Autodesk Inventor part; units mm, degrees
(part 4 of 6)
  line L840 (29.0828, -25.8646) -> (29.0171, -26.0875) projected
  line L841 (29.1718, -25.6412) -> (29.0828, -25.8646) projected
  line L842 (29.3021, -25.4012) -> (29.1718, -25.6412) projected
  line L843 (29.5054, -25.1196) -> (29.3021, -25.4012) projected
  line L844 (29.5412, -25.0774) -> (29.5054, -25.1196) projected
  line L845 (29.5771, -25.0351) -> (29.5412, -25.0774) projected
  line L846 (29.6129, -24.9928) -> (29.5771, -25.0351) projected
  line L847 (29.6486, -24.9504) -> (29.6129, -24.9928) projected
  line L848 (29.6842, -24.908) -> (29.6486, -24.9504) projected
  line L849 (29.7198, -24.8655) -> (29.6842, -24.908) projected
  line L850 (29.7553, -24.823) -> (29.7198, -24.8655) projected
  line L851 (29.7908, -24.7804) -> (29.7553, -24.823) projected
  line L852 (29.8262, -24.7378) -> (29.7908, -24.7804) projected
  line L853 (29.8616, -24.6951) -> (29.8262, -24.7378) projected
  line L854 (30.1036, -24.4461) -> (29.8616, -24.6951) projected
  line L855 (30.3173, -24.2761) -> (30.1036, -24.4461) projected
  line L856 (30.5219, -24.1496) -> (30.3173, -24.2761) projected
  line L857 (30.7299, -24.0462) -> (30.5219, -24.1496) projected
  line L858 (30.9366, -23.9692) -> (30.7299, -24.0462) projected
  line L859 (31.1483, -23.9085) -> (30.9366, -23.9692) projected
  line L860 (31.3597, -23.8696) -> (31.1483, -23.9085) projected
  line L861 (31.575, -23.8461) -> (31.3597, -23.8696) projected
  line L862 (31.7918, -23.8401) -> (31.575, -23.8461) projected
  line L863 (32.0092, -23.8521) -> (31.7918, -23.8401) projected
  line L864 (32.231, -23.8765) -> (32.0092, -23.8521) projected
  line L865 (32.4525, -23.9189) -> (32.231, -23.8765) projected
  line L866 (32.6748, -23.9775) -> (32.4525, -23.9189) projected
  line L867 (32.9013, -24.0471) -> (32.6748, -23.9775) projected
  line L868 (33.1282, -24.1326) -> (32.9013, -24.0471) projected
  line L869 (33.3555, -24.2337) -> (33.1282, -24.1326) projected
  line L870 (33.583, -24.3502) -> (33.3555, -24.2337) projected
  line L871 (33.814, -24.4773) -> (33.583, -24.3502) projected
  line L872 (34.0465, -24.6174) -> (33.814, -24.4773) projected
  line L873 (34.2792, -24.772) -> (34.0465, -24.6174) projected
  line L874 (34.6041, -24.9642) -> (34.2792, -24.772) projected
  line L875 (34.9452, -25.1339) -> (34.6041, -24.9642) projected
  line L876 (35.2972, -25.2883) -> (34.9452, -25.1339) projected
  line L877 (35.6581, -25.4299) -> (35.2972, -25.2883) projected
  line L878 (36.0268, -25.5601) -> (35.6581, -25.4299) projected
  line L879 (36.4025, -25.68) -> (36.0268, -25.5601) projected
  line L880 (36.7847, -25.7901) -> (36.4025, -25.68) projected
  line L881 (37.1729, -25.8909) -> (36.7847, -25.7901) projected
  line L882 (37.5667, -25.9828) -> (37.1729, -25.8909) projected
  line L883 (37.9659, -26.0661) -> (37.5667, -25.9828) projected
  line L884 (38.3701, -26.1411) -> (37.9659, -26.0661) projected
  line L885 (38.7791, -26.2078) -> (38.3701, -26.1411) projected
  line L886 (39.1928, -26.2665) -> (38.7791, -26.2078) projected
  line L887 (39.6108, -26.3174) -> (39.1928, -26.2665) projected
  line L888 (40.0331, -26.3604) -> (39.6108, -26.3174) projected
  line L889 (40.4594, -26.3957) -> (40.0331, -26.3604) projected
  line L890 (40.8897, -26.4234) -> (40.4594, -26.3957) projected
  line L891 (41.3237, -26.4435) -> (40.8897, -26.4234) projected
  line L892 (41.7614, -26.4561) -> (41.3237, -26.4435) projected
  line L893 (42.2025, -26.4613) -> (41.7614, -26.4561) projected
  line L894 (42.3943, -26.153) -> (42.2025, -26.4613) projected
  line L895 (42.5838, -25.8433) -> (42.3943, -26.153) projected
  line L896 (42.771, -25.5322) -> (42.5838, -25.8433) projected
  line L897 (42.9559, -25.2198) -> (42.771, -25.5322) projected
  line L898 (43.1386, -24.9061) -> (42.9559, -25.2198) projected
  line L899 (43.319, -24.591) -> (43.1386, -24.9061) projected
  line L900 (43.4971, -24.2746) -> (43.319, -24.591) projected
  line L901 (43.6728, -23.957) -> (43.4971, -24.2746) projected
  line L902 (43.8463, -23.638) -> (43.6728, -23.957) projected
  line L903 (44.0174, -23.3178) -> (43.8463, -23.638) projected
  line L904 (43.7924, -22.9383) -> (44.0174, -23.3178) projected
  line L905 (43.5626, -22.5656) -> (43.7924, -22.9383) projected
  line L906 (43.3282, -22.1998) -> (43.5626, -22.5656) projected
  line L907 (43.0891, -21.841) -> (43.3282, -22.1998) projected
  line L908 (42.8453, -21.4895) -> (43.0891, -21.841) projected
  line L909 (42.5969, -21.1453) -> (42.8453, -21.4895) projected
  line L910 (42.3439, -20.8086) -> (42.5969, -21.1453) projected
  line L911 (42.0862, -20.4798) -> (42.3439, -20.8086) projected
  line L912 (41.8239, -20.1589) -> (42.0862, -20.4798) projected
  line L913 (41.5569, -19.8464) -> (41.8239, -20.1589) projected
  line L914 (41.2851, -19.5423) -> (41.5569, -19.8464) projected
  line L915 (41.0086, -19.2472) -> (41.2851, -19.5423) projected
  line L916 (40.7272, -18.9615) -> (41.0086, -19.2472) projected
  line L917 (40.4408, -18.6855) -> (40.7272, -18.9615) projected
  line L918 (40.1491, -18.4201) -> (40.4408, -18.6855) projected
  line L919 (39.852, -18.1659) -> (40.1491, -18.4201) projected
  line L920 (39.5489, -17.9241) -> (39.852, -18.1659) projected
  line L921 (39.2392, -17.6965) -> (39.5489, -17.9241) projected
  line L922 (38.9217, -17.4859) -> (39.2392, -17.6965) projected
  line L923 (38.5928, -17.3007) -> (38.9217, -17.4859) projected
  line L924 (38.3425, -17.1764) -> (38.5928, -17.3007) projected
  line L925 (38.105, -17.0451) -> (38.3425, -17.1764) projected
  line L926 (37.8794, -16.9086) -> (38.105, -17.0451) projected
  line L927 (37.6648, -16.7698) -> (37.8794, -16.9086) projected
  line L928 (37.4636, -16.6236) -> (37.6648, -16.7698) projected
  line L929 (37.2761, -16.4698) -> (37.4636, -16.6236) projected
  line L930 (37.1025, -16.3084) -> (37.2761, -16.4698) projected
  line L931 (36.9406, -16.1452) -> (37.1025, -16.3084) projected
  line L932 (36.7931, -15.9746) -> (36.9406, -16.1452) projected
  line L933 (36.6611, -15.7947) -> (36.7931, -15.9746) projected
  line L934 (36.5421, -15.6124) -> (36.6611, -15.7947) projected
  line L935 (36.4388, -15.4218) -> (36.5421, -15.6124) projected
  line L936 (36.3516, -15.2235) -> (36.4388, -15.4218) projected
  line L937 (36.2795, -15.0209) -> (36.3516, -15.2235) projected
  line L938 (36.2262, -14.8073) -> (36.2795, -15.0209) projected
  line L939 (36.1896, -14.5898) -> (36.2262, -14.8073) projected
  line L940 (36.1751, -14.3579) -> (36.1896, -14.5898) projected
  line L941 (36.1824, -14.1175) -> (36.1751, -14.3579) projected
  line L942 (36.2227, -13.8474) -> (36.1824, -14.1175) projected
  line L943 (36.3174, -13.5133) -> (36.2227, -13.8474) projected
  line L944 (36.3367, -13.4614) -> (36.3174, -13.5133) projected
  line L945 (36.3559, -13.4094) -> (36.3367, -13.4614) projected
  line L946 (36.375, -13.3574) -> (36.3559, -13.4094) projected
  line L947 (36.3941, -13.3053) -> (36.375, -13.3574) projected
  line L948 (36.4131, -13.2533) -> (36.3941, -13.3053) projected
  line L949 (36.432, -13.2012) -> (36.4131, -13.2533) projected
  line L950 (36.4508, -13.1491) -> (36.432, -13.2012) projected
  line L951 (36.4696, -13.0969) -> (36.4508, -13.1491) projected
  line L952 (36.4883, -13.0448) -> (36.4696, -13.0969) projected
  line L953 (36.5069, -12.9926) -> (36.4883, -13.0448) projected
  line L954 (36.6492, -12.6758) -> (36.5069, -12.9926) projected
  line L955 (36.7919, -12.4429) -> (36.6492, -12.6758) projected
  line L956 (36.9408, -12.2541) -> (36.7919, -12.4429) projected
  line L957 (37.1009, -12.0858) -> (36.9408, -12.2541) projected
  line L958 (37.2688, -11.9427) -> (37.1009, -12.0858) projected
  line L959 (37.447, -11.8133) -> (37.2688, -11.9427) projected
  line L960 (37.6324, -11.7044) -> (37.447, -11.8133) projected
  line L961 (37.8267, -11.6087) -> (37.6324, -11.7044) projected
  line L962 (38.0283, -11.529) -> (37.8267, -11.6087) projected
  line L963 (38.2367, -11.4659) -> (38.0283, -11.529) projected
  line L964 (38.4534, -11.4129) -> (38.2367, -11.4659) projected
  line L965 (38.6761, -11.377) -> (38.4534, -11.4129) projected
  line L966 (38.905, -11.3561) -> (38.6761, -11.377) projected
  line L967 (39.1417, -11.344) -> (38.905, -11.3561) projected
  line L968 (39.3842, -11.3467) -> (39.1417, -11.344) projected
  line L969 (39.6323, -11.364) -> (39.3842, -11.3467) projected
  line L970 (39.886, -11.3956) -> (39.6323, -11.364) projected
  line L971 (40.1465, -11.4361) -> (39.886, -11.3956) projected
  line L972 (40.4129, -11.4882) -> (40.1465, -11.4361) projected
  line L973 (40.6845, -11.5538) -> (40.4129, -11.4882) projected
  line L974 (41.0555, -11.6234) -> (40.6845, -11.5538) projected
  line L975 (41.4341, -11.6662) -> (41.0555, -11.6234) projected
  line L976 (41.8176, -11.6908) -> (41.4341, -11.6662) projected
  line L977 (42.2052, -11.7005) -> (41.8176, -11.6908) projected
  line L978 (42.5962, -11.6968) -> (42.2052, -11.7005) projected
  line L979 (42.9903, -11.6809) -> (42.5962, -11.6968) projected
  line L980 (43.387, -11.6536) -> (42.9903, -11.6809) projected
  line L981 (43.7863, -11.6156) -> (43.387, -11.6536) projected
  line L982 (44.1878, -11.5673) -> (43.7863, -11.6156) projected
  line L983 (44.5914, -11.509) -> (44.1878, -11.5673) projected
  line L984 (44.9969, -11.4412) -> (44.5914, -11.509) projected
  line L985 (45.4041, -11.3641) -> (44.9969, -11.4412) projected
  line L986 (45.8128, -11.2778) -> (45.4041, -11.3641) projected
  line L987 (46.223, -11.1825) -> (45.8128, -11.2778) projected
  line L988 (46.6346, -11.0786) -> (46.223, -11.1825) projected
  line L989 (47.0473, -10.9659) -> (46.6346, -11.0786) projected
  line L990 (47.4611, -10.8448) -> (47.0473, -10.9659) projected
  line L991 (47.8758, -10.7152) -> (47.4611, -10.8448) projected
  line L992 (48.2914, -10.5774) -> (47.8758, -10.7152) projected
  line L993 (48.7077, -10.4313) -> (48.2914, -10.5774) projected
  line L994 (48.7824, -10.0761) -> (48.7077, -10.4313) projected
  line L995 (48.8546, -9.7203) -> (48.7824, -10.0761) projected
  line L996 (48.9241, -9.3639) -> (48.8546, -9.7203) projected
  line L997 (48.9911, -9.0071) -> (48.9241, -9.3639) projected
  line L998 (49.0554, -8.6498) -> (48.9911, -9.0071) projected
  line L999 (49.1172, -8.292) -> (49.0554, -8.6498) projected
  line L1000 (49.1763, -7.9338) -> (49.1172, -8.292) projected
  line L1001 (49.2328, -7.5752) -> (49.1763, -7.9338) projected
  line L1002 (49.2867, -7.2162) -> (49.2328, -7.5752) projected
  line L1003 (49.338, -6.8568) -> (49.2867, -7.2162) projected
  line L1004 (48.9968, -6.5771) -> (49.338, -6.8568) projected
  line L1005 (48.6534, -6.3055) -> (48.9968, -6.5771) projected
  line L1006 (48.308, -6.0419) -> (48.6534, -6.3055) projected
  line L1007 (47.9606, -5.7865) -> (48.308, -6.0419) projected
  line L1008 (47.6113, -5.5395) -> (47.9606, -5.7865) projected
  line L1009 (47.2601, -5.3011) -> (47.6113, -5.5395) projected
  line L1010 (46.9072, -5.0713) -> (47.2601, -5.3011) projected
  line L1011 (46.5526, -4.8504) -> (46.9072, -5.0713) projected
  line L1012 (46.1963, -4.6386) -> (46.5526, -4.8504) projected
  line L1013 (45.8385, -4.4362) -> (46.1963, -4.6386) projected
  line L1014 (45.4792, -4.2434) -> (45.8385, -4.4362) projected
  line L1015 (45.1184, -4.0607) -> (45.4792, -4.2434) projected
  line L1016 (44.7563, -3.8884) -> (45.1184, -4.0607) projected
  line L1017 (44.3927, -3.7271) -> (44.7563, -3.8884) projected
  line L1018 (44.0279, -3.5774) -> (44.3927, -3.7271) projected
  line L1019 (43.6617, -3.4402) -> (44.0279, -3.5774) projected
  line L1020 (43.2942, -3.3167) -> (43.6617, -3.4402) projected
  line L1021 (42.9254, -3.2087) -> (43.2942, -3.3167) projected
  line L1022 (42.555, -3.1194) -> (42.9254, -3.2087) projected
  line L1023 (42.1825, -3.0578) -> (42.555, -3.1194) projected
  line L1024 (41.9049, -3.0266) -> (42.1825, -3.0578) projected
  line L1025 (41.6367, -2.9845) -> (41.9049, -3.0266) projected
  line L1026 (41.3781, -2.9334) -> (41.6367, -2.9845) projected
  line L1027 (41.1289, -2.8764) -> (41.3781, -2.9334) projected
  line L1028 (40.8898, -2.8078) -> (41.1289, -2.8764) projected
  line L1029 (40.661, -2.7274) -> (40.8898, -2.8078) projected
  line L1030 (40.4428, -2.6351) -> (40.661, -2.7274) projected
  line L1031 (40.2348, -2.5371) -> (40.4428, -2.6351) projected
  line L1032 (40.0379, -2.4272) -> (40.2348, -2.5371) projected
  line L1033 (39.8523, -2.3033) -> (40.0379, -2.4272) projected
  line L1034 (39.6781, -2.1727) -> (39.8523, -2.3033) projected
  line L1035 (39.5158, -2.0289) -> (39.6781, -2.1727) projected
  line L1036 (39.366, -1.8725) -> (39.5158, -2.0289) projected
  line L1037 (39.2291, -1.7067) -> (39.366, -1.8725) projected
  line L1038 (39.1059, -1.5242) -> (39.2291, -1.7067) projected
  line L1039 (38.997, -1.3323) -> (39.1059, -1.5242) projected
  line L1040 (38.9042, -1.1194) -> (38.997, -1.3323) projected
  line L1041 (38.8288, -0.891) -> (38.9042, -1.1194) projected
  line L1042 (38.7743, -0.6234) -> (38.8288, -0.891) projected
  line L1043 (38.749, -0.2771) -> (38.7743, -0.6234) projected
  line L1044 (38.7494, -0.2217) -> (38.749, -0.2771) projected
  line L1045 (38.7496, -0.1663) -> (38.7494, -0.2217) projected
  line L1046 (38.7498, -0.1108) -> (38.7496, -0.1663) projected
  line L1047 (38.75, -0.0554) -> (38.7498, -0.1108) projected
  line L1048 (38.75, 0) -> (38.75, -0.0554) projected
  line L1049 (38.75, 0.0554) -> (38.75, 0) projected
  line L1050 (38.7498, 0.1108) -> (38.75, 0.0554) projected
  line L1051 (38.7496, 0.1663) -> (38.7498, 0.1108) projected
  line L1052 (38.7494, 0.2217) -> (38.7496, 0.1663) projected
  line L1053 (38.749, 0.2771) -> (38.7494, 0.2217) projected
  line L1054 (38.7743, 0.6234) -> (38.749, 0.2771) projected
  line L1055 (38.8288, 0.891) -> (38.7743, 0.6234) projected
  line L1056 (38.9042, 1.1194) -> (38.8288, 0.891) projected
  line L1057 (38.997, 1.3323) -> (38.9042, 1.1194) projected
  line L1058 (39.1059, 1.5242) -> (38.997, 1.3323) projected
  line L1059 (39.2291, 1.7067) -> (39.1059, 1.5242) projected
  line L1060 (39.366, 1.8725) -> (39.2291, 1.7067) projected
  line L1061 (39.5158, 2.0289) -> (39.366, 1.8725) projected
  line L1062 (39.6781, 2.1727) -> (39.5158, 2.0289) projected
  line L1063 (39.8523, 2.3033) -> (39.6781, 2.1727) projected
  line L1064 (40.0379, 2.4272) -> (39.8523, 2.3033) projected
  line L1065 (40.2348, 2.5371) -> (40.0379, 2.4272) projected
  line L1066 (40.4428, 2.6351) -> (40.2348, 2.5371) projected
  line L1067 (40.661, 2.7274) -> (40.4428, 2.6351) projected
  line L1068 (40.8898, 2.8078) -> (40.661, 2.7274) projected
  line L1069 (41.1289, 2.8764) -> (40.8898, 2.8078) projected
  line L1070 (41.3781, 2.9334) -> (41.1289, 2.8764) projected
  line L1071 (41.6367, 2.9845) -> (41.3781, 2.9334) projected
  line L1072 (41.9049, 3.0266) -> (41.6367, 2.9845) projected
  line L1073 (42.1825, 3.0578) -> (41.9049, 3.0266) projected
  line L1074 (42.555, 3.1194) -> (42.1825, 3.0578) projected
  line L1075 (42.9254, 3.2087) -> (42.555, 3.1194) projected
  line L1076 (43.2942, 3.3167) -> (42.9254, 3.2087) projected
  line L1077 (43.6617, 3.4402) -> (43.2942, 3.3167) projected
  line L1078 (44.0279, 3.5774) -> (43.6617, 3.4402) projected
  line L1079 (44.3927, 3.7271) -> (44.0279, 3.5774) projected
  line L1080 (44.7563, 3.8884) -> (44.3927, 3.7271) projected
  line L1081 (45.1184, 4.0607) -> (44.7563, 3.8884) projected
  line L1082 (45.4792, 4.2434) -> (45.1184, 4.0607) projected
  line L1083 (45.8385, 4.4362) -> (45.4792, 4.2434) projected
  line L1084 (46.1963, 4.6386) -> (45.8385, 4.4362) projected
  line L1085 (46.5526, 4.8504) -> (46.1963, 4.6386) projected
  line L1086 (46.9072, 5.0713) -> (46.5526, 4.8504) projected
  line L1087 (47.2601, 5.3011) -> (46.9072, 5.0713) projected
  line L1088 (47.6113, 5.5395) -> (47.2601, 5.3011) projected
  line L1089 (47.9606, 5.7865) -> (47.6113, 5.5395) projected
  line L1090 (48.308, 6.0419) -> (47.9606, 5.7865) projected
  line L1091 (48.6534, 6.3055) -> (48.308, 6.0419) projected
  line L1092 (48.9968, 6.5771) -> (48.6534, 6.3055) projected
  line L1093 (49.338, 6.8568) -> (48.9968, 6.5771) projected
  line L1094 (49.2867, 7.2162) -> (49.338, 6.8568) projected
  line L1095 (49.2328, 7.5752) -> (49.2867, 7.2162) projected
  line L1096 (49.1763, 7.9338) -> (49.2328, 7.5752) projected
  line L1097 (49.1172, 8.292) -> (49.1763, 7.9338) projected
  line L1098 (49.0554, 8.6498) -> (49.1172, 8.292) projected
  line L1099 (48.9911, 9.0071) -> (49.0554, 8.6498) projected
  line L1100 (48.9241, 9.3639) -> (48.9911, 9.0071) projected
  line L1101 (48.8546, 9.7203) -> (48.9241, 9.3639) projected
  line L1102 (48.7824, 10.0761) -> (48.8546, 9.7203) projected
  line L1103 (48.7077, 10.4313) -> (48.7824, 10.0761) projected
  line L1104 (48.2914, 10.5774) -> (48.7077, 10.4313) projected
  line L1105 (47.8758, 10.7152) -> (48.2914, 10.5774) projected
  line L1106 (47.4611, 10.8448) -> (47.8758, 10.7152) projected
  line L1107 (47.0473, 10.9659) -> (47.4611, 10.8448) projected
  line L1108 (46.6346, 11.0786) -> (47.0473, 10.9659) projected
  line L1109 (46.223, 11.1825) -> (46.6346, 11.0786) projected
  line L1110 (45.8128, 11.2778) -> (46.223, 11.1825) projected
  line L1111 (45.4041, 11.3641) -> (45.8128, 11.2778) projected
  line L1112 (44.9969, 11.4412) -> (45.4041, 11.3641) projected
  line L1113 (44.5914, 11.509) -> (44.9969, 11.4412) projected
  line L1114 (44.1878, 11.5673) -> (44.5914, 11.509) projected
  line L1115 (43.7863, 11.6156) -> (44.1878, 11.5673) projected
  line L1116 (43.387, 11.6536) -> (43.7863, 11.6156) projected
  line L1117 (42.9903, 11.6809) -> (43.387, 11.6536) projected
  line L1118 (42.5962, 11.6968) -> (42.9903, 11.6809) projected
  line L1119 (42.2052, 11.7005) -> (42.5962, 11.6968) projected
  line L1120 (41.8176, 11.6908) -> (42.2052, 11.7005) projected
  line L1121 (41.4341, 11.6662) -> (41.8176, 11.6908) projected
  line L1122 (41.0555, 11.6234) -> (41.4341, 11.6662) projected
  line L1123 (40.6845, 11.5538) -> (41.0555, 11.6234) projected
  line L1124 (40.4129, 11.4882) -> (40.6845, 11.5538) projected
  line L1125 (40.1465, 11.4361) -> (40.4129, 11.4882) projected
  line L1126 (39.886, 11.3956) -> (40.1465, 11.4361) projected
  line L1127 (39.6323, 11.364) -> (39.886, 11.3956) projected
  line L1128 (39.3842, 11.3467) -> (39.6323, 11.364) projected
  line L1129 (39.1417, 11.344) -> (39.3842, 11.3467) projected
  line L1130 (38.905, 11.3561) -> (39.1417, 11.344) projected
  line L1131 (38.6761, 11.377) -> (38.905, 11.3561) projected
  line L1132 (38.4534, 11.4129) -> (38.6761, 11.377) projected
  line L1133 (38.2367, 11.4659) -> (38.4534, 11.4129) projected
  line L1134 (38.0283, 11.529) -> (38.2367, 11.4659) projected
  line L1135 (37.8267, 11.6087) -> (38.0283, 11.529) projected
  line L1136 (37.6324, 11.7044) -> (37.8267, 11.6087) projected
  line L1137 (37.447, 11.8133) -> (37.6324, 11.7044) projected
  line L1138 (37.2688, 11.9427) -> (37.447, 11.8133) projected
  line L1139 (37.1009, 12.0858) -> (37.2688, 11.9427) projected
  line L1140 (36.9408, 12.2541) -> (37.1009, 12.0858) projected
  line L1141 (36.7919, 12.4429) -> (36.9408, 12.2541) projected
  line L1142 (36.6492, 12.6758) -> (36.7919, 12.4429) projected
  line L1143 (36.5069, 12.9926) -> (36.6492, 12.6758) projected
  line L1144 (36.4883, 13.0448) -> (36.5069, 12.9926) projected
  line L1145 (36.4696, 13.0969) -> (36.4883, 13.0448) projected
  line L1146 (36.4508, 13.1491) -> (36.4696, 13.0969) projected
  line L1147 (36.432, 13.2012) -> (36.4508, 13.1491) projected
  line L1148 (36.4131, 13.2533) -> (36.432, 13.2012) projected
  line L1149 (36.3941, 13.3053) -> (36.4131, 13.2533) projected
  line L1150 (36.375, 13.3574) -> (36.3941, 13.3053) projected
  line L1151 (36.3559, 13.4094) -> (36.375, 13.3574) projected
  line L1152 (36.3367, 13.4614) -> (36.3559, 13.4094) projected
  line L1153 (36.3174, 13.5133) -> (36.3367, 13.4614) projected
  line L1154 (36.2227, 13.8474) -> (36.3174, 13.5133) projected
  line L1155 (36.1824, 14.1175) -> (36.2227, 13.8474) projected
  line L1156 (36.1751, 14.3579) -> (36.1824, 14.1175) projected
  line L1157 (36.1896, 14.5898) -> (36.1751, 14.3579) projected
  line L1158 (36.2262, 14.8073) -> (36.1896, 14.5898) projected
  line L1159 (36.2795, 15.0209) -> (36.2262, 14.8073) projected
  line L1160 (36.3516, 15.2235) -> (36.2795, 15.0209) projected
  line L1161 (36.4388, 15.4218) -> (36.3516, 15.2235) projected
  line L1162 (36.5421, 15.6124) -> (36.4388, 15.4218) projected
  line L1163 (36.6611, 15.7947) -> (36.5421, 15.6124) projected
  line L1164 (36.7931, 15.9746) -> (36.6611, 15.7947) projected
  line L1165 (36.9406, 16.1452) -> (36.7931, 15.9746) projected
  line L1166 (37.1025, 16.3084) -> (36.9406, 16.1452) projected
  line L1167 (37.2761, 16.4698) -> (37.1025, 16.3084) projected
  line L1168 (37.4636, 16.6236) -> (37.2761, 16.4698) projected
  line L1169 (37.6648, 16.7698) -> (37.4636, 16.6236) projected
  line L1170 (37.8794, 16.9086) -> (37.6648, 16.7698) projected
  line L1171 (38.105, 17.0451) -> (37.8794, 16.9086) projected
  line L1172 (38.3425, 17.1764) -> (38.105, 17.0451) projected
  line L1173 (38.5928, 17.3007) -> (38.3425, 17.1764) projected
  line L1174 (38.9217, 17.4859) -> (38.5928, 17.3007) projected
  line L1175 (39.2392, 17.6965) -> (38.9217, 17.4859) projected
  line L1176 (39.5489, 17.9241) -> (39.2392, 17.6965) projected
  line L1177 (39.852, 18.1659) -> (39.5489, 17.9241) projected
  line L1178 (40.1491, 18.4201) -> (39.852, 18.1659) projected
  line L1179 (40.4408, 18.6855) -> (40.1491, 18.4201) projected
  line L1180 (40.7272, 18.9615) -> (40.4408, 18.6855) projected
  line L1181 (41.0086, 19.2472) -> (40.7272, 18.9615) projected
  line L1182 (41.2851, 19.5423) -> (41.0086, 19.2472) projected
  line L1183 (41.5569, 19.8464) -> (41.2851, 19.5423) projected
  line L1184 (41.8239, 20.1589) -> (41.5569, 19.8464) projected
  line L1185 (42.0862, 20.4798) -> (41.8239, 20.1589) projected
  line L1186 (42.3439, 20.8086) -> (42.0862, 20.4798) projected
  line L1187 (42.5969, 21.1453) -> (42.3439, 20.8086) projected
  line L1188 (42.8453, 21.4895) -> (42.5969, 21.1453) projected
  line L1189 (43.0891, 21.841) -> (42.8453, 21.4895) projected
  line L1190 (43.3282, 22.1998) -> (43.0891, 21.841) projected
  line L1191 (43.5626, 22.5656) -> (43.3282, 22.1998) projected
  line L1192 (43.7924, 22.9383) -> (43.5626, 22.5656) projected
  line L1193 (44.0174, 23.3178) -> (43.7924, 22.9383) projected
  line L1194 (43.8463, 23.638) -> (44.0174, 23.3178) projected
  line L1195 (43.6728, 23.957) -> (43.8463, 23.638) projected
  line L1196 (43.4971, 24.2746) -> (43.6728, 23.957) projected
  line L1197 (43.319, 24.591) -> (43.4971, 24.2746) projected
  line L1198 (43.1386, 24.9061) -> (43.319, 24.591) projected
  line L1199 (42.9559, 25.2198) -> (43.1386, 24.9061) projected
  line L1200 (42.771, 25.5322) -> (42.9559, 25.2198) projected
  line L1201 (42.5838, 25.8433) -> (42.771, 25.5322) projected
  line L1202 (42.3943, 26.153) -> (42.5838, 25.8433) projected
  line L1203 (42.2025, 26.4613) -> (42.3943, 26.153) projected
  line L1204 (41.7614, 26.4561) -> (42.2025, 26.4613) projected
  line L1205 (41.3237, 26.4435) -> (41.7614, 26.4561) projected
  line L1206 (40.8897, 26.4234) -> (41.3237, 26.4435) projected
  line L1207 (40.4594, 26.3957) -> (40.8897, 26.4234) projected
  line L1208 (40.0331, 26.3604) -> (40.4594, 26.3957) projected
  line L1209 (39.6108, 26.3174) -> (40.0331, 26.3604) projected
  line L1210 (39.1928, 26.2665) -> (39.6108, 26.3174) projected
  line L1211 (38.7791, 26.2078) -> (39.1928, 26.2665) projected
  line L1212 (38.3701, 26.1411) -> (38.7791, 26.2078) projected
  line L1213 (37.9659, 26.0661) -> (38.3701, 26.1411) projected
  line L1214 (37.5667, 25.9828) -> (37.9659, 26.0661) projected
  line L1215 (37.1729, 25.8909) -> (37.5667, 25.9828) projected
  line L1216 (36.7847, 25.7901) -> (37.1729, 25.8909) projected
  line L1217 (36.4025, 25.68) -> (36.7847, 25.7901) projected
  line L1218 (36.0268, 25.5601) -> (36.4025, 25.68) projected
  line L1219 (35.6581, 25.4299) -> (36.0268, 25.5601) projected
  line L1220 (35.2972, 25.2883) -> (35.6581, 25.4299) projected
  line L1221 (34.9452, 25.1339) -> (35.2972, 25.2883) projected
  line L1222 (34.6041, 24.9642) -> (34.9452, 25.1339) projected
  line L1223 (34.2792, 24.772) -> (34.6041, 24.9642) projected
  line L1224 (34.0465, 24.6174) -> (34.2792, 24.772) projected
  line L1225 (33.814, 24.4773) -> (34.0465, 24.6174) projected
  line L1226 (33.583, 24.3502) -> (33.814, 24.4773) projected
  line L1227 (33.3555, 24.2337) -> (33.583, 24.3502) projected
  line L1228 (33.1282, 24.1326) -> (33.3555, 24.2337) projected
  line L1229 (32.9013, 24.0471) -> (33.1282, 24.1326) projected
  line L1230 (32.6748, 23.9775) -> (32.9013, 24.0471) projected
  line L1231 (32.4525, 23.9189) -> (32.6748, 23.9775) projected
  line L1232 (32.231, 23.8765) -> (32.4525, 23.9189) projected
  line L1233 (32.0092, 23.8521) -> (32.231, 23.8765) projected
  line L1234 (31.7918, 23.8401) -> (32.0092, 23.8521) projected
  line L1235 (31.575, 23.8461) -> (31.7918, 23.8401) projected
  line L1236 (31.3597, 23.8696) -> (31.575, 23.8461) projected
  line L1237 (31.1483, 23.9085) -> (31.3597, 23.8696) projected
  line L1238 (30.9366, 23.9692) -> (31.1483, 23.9085) projected
  line L1239 (30.7299, 24.0462) -> (30.9366, 23.9692) projected
  line L1240 (30.5219, 24.1496) -> (30.7299, 24.0462) projected
  line L1241 (30.3173, 24.2761) -> (30.5219, 24.1496) projected
  line L1242 (30.1036, 24.4461) -> (30.3173, 24.2761) projected
  line L1243 (29.8616, 24.6951) -> (30.1036, 24.4461) projected
  line L1244 (29.8262, 24.7378) -> (29.8616, 24.6951) projected
  line L1245 (29.7908, 24.7804) -> (29.8262, 24.7378) projected
  line L1246 (29.7553, 24.823) -> (29.7908, 24.7804) projected
  line L1247 (29.7198, 24.8655) -> (29.7553, 24.823) projected
  line L1248 (29.6842, 24.908) -> (29.7198, 24.8655) projected
  line L1249 (29.6486, 24.9504) -> (29.6842, 24.908) projected
  line L1250 (29.6129, 24.9928) -> (29.6486, 24.9504) projected
  line L1251 (29.5771, 25.0351) -> (29.6129, 24.9928) projected
  line L1252 (29.5412, 25.0774) -> (29.5771, 25.0351) projected
  line L1253 (29.5054, 25.1196) -> (29.5412, 25.0774) projected
  line L1254 (29.3021, 25.4012) -> (29.5054, 25.1196) projected
  line L1255 (29.1718, 25.6412) -> (29.3021, 25.4012) projected
  line L1256 (29.0828, 25.8646) -> (29.1718, 25.6412) projected
  line L1257 (29.0171, 26.0875) -> (29.0828, 25.8646) projected
  line L1258 (28.9771, 26.3044) -> (29.0171, 26.0875) projected
  line L1259 (28.9541, 26.5234) -> (28.9771, 26.3044) projected
  line L1260 (28.9525, 26.7384) -> (28.9541, 26.5234) projected
  line L1261 (28.9667, 26.9545) -> (28.9525, 26.7384) projected
  line L1262 (28.9985, 27.169) -> (28.9667, 26.9545) projected
  line L1263 (29.0481, 27.381) -> (28.9985, 27.169) projected
  line L1264 (29.1106, 27.5952) -> (29.0481, 27.381) projected
  line L1265 (29.1908, 27.806) -> (29.1106, 27.5952) projected
  line L1266 (29.2872, 28.0147) -> (29.1908, 27.806) projected
  line L1267 (29.395, 28.2257) -> (29.2872, 28.0147) projected
  line L1268 (29.5186, 28.4343) -> (29.395, 28.2257) projected
  line L1269 (29.6577, 28.6406) -> (29.5186, 28.4343) projected
  line L1270 (29.8119, 28.8444) -> (29.6577, 28.6406) projected
  line L1271 (29.9772, 29.0498) -> (29.8119, 28.8444) projected
  line L1272 (30.1555, 29.2545) -> (29.9772, 29.0498) projected
  line L1273 (30.3482, 29.4569) -> (30.1555, 29.2545) projected
  line L1274 (30.5939, 29.7434) -> (30.3482, 29.4569) projected
  line L1275 (30.8202, 30.0499) -> (30.5939, 29.7434) projected
  line L1276 (31.0334, 30.3697) -> (30.8202, 30.0499) projected
  line L1277 (31.2355, 30.7005) -> (31.0334, 30.3697) projected
  line L1278 (31.4278, 31.041) -> (31.2355, 30.7005) projected
  line L1279 (31.6111, 31.3902) -> (31.4278, 31.041) projected
  line L1280 (31.7858, 31.7475) -> (31.6111, 31.3902) projected
  line L1281 (31.9525, 32.1123) -> (31.7858, 31.7475) projected
  line L1282 (32.1115, 32.4841) -> (31.9525, 32.1123) projected
  line L1283 (32.2628, 32.8628) -> (32.1115, 32.4841) projected
  line L1284 (32.4068, 33.2478) -> (32.2628, 32.8628) projected
  line L1285 (32.5436, 33.639) -> (32.4068, 33.2478) projected
  line L1286 (32.6732, 34.0362) -> (32.5436, 33.639) projected
  line L1287 (32.7959, 34.4391) -> (32.6732, 34.0362) projected
  line L1288 (32.9116, 34.8475) -> (32.7959, 34.4391) projected
  line L1289 (33.0204, 35.2612) -> (32.9116, 34.8475) projected
  line L1290 (33.1224, 35.6801) -> (33.0204, 35.2612) projected
  line L1291 (33.2176, 36.1041) -> (33.1224, 35.6801) projected
  line L1292 (33.306, 36.5329) -> (33.2176, 36.1041) projected
  line L1293 (33.3877, 36.9664) -> (33.306, 36.5329) projected
  line L1294 (33.1173, 37.2088) -> (33.3877, 36.9664) projected
  line L1295 (32.8453, 37.4492) -> (33.1173, 37.2088) projected
  line L1296 (32.5715, 37.6876) -> (32.8453, 37.4492) projected
  line L1297 (32.2959, 37.924) -> (32.5715, 37.6876) projected
  line L1298 (32.0186, 38.1583) -> (32.2959, 37.924) projected
  line L1299 (31.7397, 38.3907) -> (32.0186, 38.1583) projected
  line L1300 (31.459, 38.621) -> (31.7397, 38.3907) projected
  line L1301 (31.1767, 38.8493) -> (31.459, 38.621) projected
  line L1302 (30.8927, 39.0755) -> (31.1767, 38.8493) projected
  line L1303 (30.6071, 39.2996) -> (30.8927, 39.0755) projected
  line L1304 (30.1943, 39.1439) -> (30.6071, 39.2996) projected
  line L1305 (29.7874, 38.9823) -> (30.1943, 39.1439) projected
  line L1306 (29.3864, 38.815) -> (29.7874, 38.9823) projected
  line L1307 (28.9916, 38.6418) -> (29.3864, 38.815) projected
  line L1308 (28.603, 38.4628) -> (28.9916, 38.6418) projected
  line L1309 (28.2209, 38.2779) -> (28.603, 38.4628) projected
  line L1310 (27.8455, 38.0872) -> (28.2209, 38.2779) projected
  line L1311 (27.4768, 37.8905) -> (27.8455, 38.0872) projected
  line L1312 (27.1153, 37.6879) -> (27.4768, 37.8905) projected
  line L1313 (26.7611, 37.4792) -> (27.1153, 37.6879) projected
  line L1314 (26.4145, 37.2644) -> (26.7611, 37.4792) projected
  line L1315 (26.0759, 37.0434) -> (26.4145, 37.2644) projected
  line L1316 (25.7456, 36.8158) -> (26.0759, 37.0434) projected
  line L1317 (25.4241, 36.5817) -> (25.7456, 36.8158) projected
  line L1318 (25.1121, 36.3405) -> (25.4241, 36.5817) projected
  line L1319 (24.8101, 36.092) -> (25.1121, 36.3405) projected
  line L1320 (24.5194, 35.8356) -> (24.8101, 36.092) projected
  line L1321 (24.2415, 35.5701) -> (24.5194, 35.8356) projected
  line L1322 (23.979, 35.294) -> (24.2415, 35.5701) projected
  line L1323 (23.7394, 35.0022) -> (23.979, 35.294) projected
  line L1324 (23.5736, 34.7774) -> (23.7394, 35.0022) projected
  line L1325 (23.403, 34.5662) -> (23.5736, 34.7774) projected
  line L1326 (23.2294, 34.3678) -> (23.403, 34.5662) projected
  line L1327 (23.0555, 34.1805) -> (23.2294, 34.3678) projected
  line L1328 (22.8765, 34.0078) -> (23.0555, 34.1805) projected
  line L1329 (22.6925, 33.8498) -> (22.8765, 34.0078) projected
  line L1330 (22.5034, 33.7069) -> (22.6925, 33.8498) projected
  line L1331 (22.3146, 33.5758) -> (22.5034, 33.7069) projected
  line L1332 (22.121, 33.4602) -> (22.3146, 33.5758) projected
  line L1333 (21.9209, 33.3615) -> (22.121, 33.4602) projected
  line L1334 (21.7207, 33.2758) -> (21.9209, 33.3615) projected
  line L1335 (21.515, 33.2073) -> (21.7207, 33.2758) projected
  line L1336 (21.3046, 33.1558) -> (21.515, 33.2073) projected
  line L1337 (21.0926, 33.12) -> (21.3046, 33.1558) projected
  line L1338 (20.8729, 33.1046) -> (21.0926, 33.12) projected
  line L1339 (20.6524, 33.1063) -> (20.8729, 33.1046) projected
  line L1340 (20.4215, 33.1323) -> (20.6524, 33.1063) projected
  line L1341 (20.186, 33.1812) -> (20.4215, 33.1323) projected
  line L1342 (19.9271, 33.2679) -> (20.186, 33.1812) projected
  line L1343 (19.6145, 33.4191) -> (19.9271, 33.2679) projected
  line L1344 (19.5667, 33.4471) -> (19.6145, 33.4191) projected
  line L1345 (19.5188, 33.475) -> (19.5667, 33.4471) projected
  line L1346 (19.4709, 33.5029) -> (19.5188, 33.475) projected
  line L1347 (19.423, 33.5307) -> (19.4709, 33.5029) projected
  line L1348 (19.375, 33.5585) -> (19.423, 33.5307) projected
  line L1349 (19.327, 33.5862) -> (19.375, 33.5585) projected
  line L1350 (19.2789, 33.6138) -> (19.327, 33.5862) projected
  line L1351 (19.2308, 33.6413) -> (19.2789, 33.6138) projected
  line L1352 (19.1827, 33.6688) -> (19.2308, 33.6413) projected
  line L1353 (19.1345, 33.6962) -> (19.1827, 33.6688) projected
  line L1354 (18.8473, 33.8913) -> (19.1345, 33.6962) projected
  line L1355 (18.6427, 34.0722) -> (18.8473, 33.8913) projected
  line L1356 (18.4826, 34.2517) -> (18.6427, 34.0722) projected
  line L1357 (18.3447, 34.4386) -> (18.4826, 34.2517) projected
  line L1358 (18.2329, 34.6288) -> (18.3447, 34.4386) projected
  line L1359 (18.1365, 34.8267) -> (18.2329, 34.6288) projected
  line L1360 (18.0614, 35.0282) -> (18.1365, 34.8267) projected
  line L1361 (18.0008, 35.2362) -> (18.0614, 35.0282) projected
  line L1362 (17.9574, 35.4486) -> (18.0008, 35.2362) projected
  line L1363 (17.9314, 35.6648) -> (17.9574, 35.4486) projected
  line L1364 (17.9169, 35.8874) -> (17.9314, 35.6648) projected
  line L1365 (17.9202, 36.1129) -> (17.9169, 35.8874) projected
  line L1366 (17.9393, 36.342) -> (17.9202, 36.1129) projected
  line L1367 (17.9685, 36.5772) -> (17.9393, 36.342) projected
  line L1368 (18.0133, 36.8155) -> (17.9685, 36.5772) projected
  line L1369 (18.0734, 37.0569) -> (18.0133, 36.8155) projected
  line L1370 (18.1486, 37.3012) -> (18.0734, 37.0569) projected
  line L1371 (18.2337, 37.5507) -> (18.1486, 37.3012) projected
  line L1372 (18.3313, 37.804) -> (18.2337, 37.5507) projected
  line L1373 (18.4431, 38.0601) -> (18.3313, 37.804) projected
  line L1374 (18.576, 38.4134) -> (18.4431, 38.0601) projected
  line L1375 (18.6839, 38.7788) -> (18.576, 38.4134) projected
  line L1376 (18.7748, 39.1522) -> (18.6839, 38.7788) projected
  line L1377 (18.8516, 39.5322) -> (18.7748, 39.1522) projected
  line L1378 (18.9158, 39.9179) -> (18.8516, 39.5322) projected
  line L1379 (18.9686, 40.3088) -> (18.9158, 39.9179) projected
  line L1380 (19.0107, 40.7043) -> (18.9686, 40.3088) projected
  line L1381 (19.0425, 41.1041) -> (19.0107, 40.7043) projected
  line L1382 (19.0647, 41.5079) -> (19.0425, 41.1041) projected
  line L1383 (19.0774, 41.9154) -> (19.0647, 41.5079) projected
  line L1384 (19.081, 42.3265) -> (19.0774, 41.9154) projected
  line L1385 (19.0757, 42.7409) -> (19.081, 42.3265) projected
  line L1386 (19.0617, 43.1585) -> (19.0757, 42.7409) projected
  line L1387 (19.0392, 43.579) -> (19.0617, 43.1585) projected
  line L1388 (19.0083, 44.0023) -> (19.0392, 43.579) projected
  line L1389 (18.969, 44.4283) -> (19.0083, 44.0023) projected
  line L1390 (18.9216, 44.8569) -> (18.969, 44.4283) projected
  line L1391 (18.866, 45.2878) -> (18.9216, 44.8569) projected
  line L1392 (18.8024, 45.721) -> (18.866, 45.2878) projected
  line L1393 (18.7309, 46.1563) -> (18.8024, 45.721) projected
  line L1394 (18.394, 46.2916) -> (18.7309, 46.1563) projected
  line L1395 (18.0561, 46.4245) -> (18.394, 46.2916) projected
  line L1396 (17.7172, 46.5548) -> (18.0561, 46.4245) projected
  line L1397 (17.3775, 46.6827) -> (17.7172, 46.5548) projected
  line L1398 (17.0368, 46.8081) -> (17.3775, 46.6827) projected
  line L1399 (16.6952, 46.9311) -> (17.0368, 46.8081) projected
  line L1400 (16.3527, 47.0515) -> (16.6952, 46.9311) projected
  line L1401 (16.0093, 47.1694) -> (16.3527, 47.0515) projected
  line L1402 (15.6651, 47.2849) -> (16.0093, 47.1694) projected
  line L1403 (15.32, 47.3978) -> (15.6651, 47.2849) projected
  line L1404 (14.9854, 47.1103) -> (15.32, 47.3978) projected
  line L1405 (14.6582, 46.8193) -> (14.9854, 47.1103) projected
  line L1406 (14.3387, 46.5249) -> (14.6582, 46.8193) projected
  line L1407 (14.0269, 46.2271) -> (14.3387, 46.5249) projected
  line L1408 (13.723, 45.926) -> (14.0269, 46.2271) projected
  line L1409 (13.4272, 45.6216) -> (13.723, 45.926) projected
  line L1410 (13.1396, 45.314) -> (13.4272, 45.6216) projected
  line L1411 (12.8605, 45.0031) -> (13.1396, 45.314) projected
  line L1412 (12.59, 44.689) -> (12.8605, 45.0031) projected
  line L1413 (12.3286, 44.3718) -> (12.59, 44.689) projected
  line L1414 (12.0764, 44.0514) -> (12.3286, 44.3718) projected
  line L1415 (11.8338, 43.7278) -> (12.0764, 44.0514) projected
  line L1416 (11.6012, 43.4011) -> (11.8338, 43.7278) projected
  line L1417 (11.3792, 43.0711) -> (11.6012, 43.4011) projected
  line L1418 (11.1684, 42.7378) -> (11.3792, 43.0711) projected
  line L1419 (10.9697, 42.401) -> (11.1684, 42.7378) projected
  line L1420 (10.7842, 42.0605) -> (10.9697, 42.401) projected
  line L1421 (10.6138, 41.716) -> (10.7842, 42.0605) projected
  line L1422 (10.4616, 41.3668) -> (10.6138, 41.716) projected
  line L1423 (10.3363, 41.0107) -> (10.4616, 41.3668) projected
  line L1424 (10.2574, 40.7427) -> (10.3363, 41.0107) projected
  line L1425 (10.1693, 40.4859) -> (10.2574, 40.7427) projected
  line L1426 (10.0741, 40.2401) -> (10.1693, 40.4859) projected
  line L1427 (9.9747, 40.0046) -> (10.0741, 40.2401) projected
  line L1428 (9.8655, 39.7811) -> (9.9747, 40.0046) projected
  line L1429 (9.7467, 39.5697) -> (9.8655, 39.7811) projected
  line L1430 (9.6179, 39.3708) -> (9.7467, 39.5697) projected
  line L1431 (9.4853, 39.183) -> (9.6179, 39.3708) projected
  line L1432 (9.3428, 39.0081) -> (9.4853, 39.183) projected
  line L1433 (9.1886, 38.8469) -> (9.3428, 39.0081) projected
  line L1434 (9.0298, 38.698) -> (9.1886, 38.8469) projected
  line L1435 (8.8599, 38.5632) -> (9.0298, 38.698) projected
  line L1436 (8.6799, 38.4428) -> (8.8599, 38.5632) projected
  line L1437 (8.4928, 38.3367) -> (8.6799, 38.4428) projected
  line L1438 (8.2917, 38.2471) -> (8.4928, 38.3367) projected
  line L1439 (8.0839, 38.1732) -> (8.2917, 38.2471) projected
  line L1440 (7.8581, 38.1187) -> (8.0839, 38.1732) projected
  line L1441 (7.62, 38.0842) -> (7.8581, 38.1187) projected
  line L1442 (7.347, 38.077) -> (7.62, 38.0842) projected
  line L1443 (7.0016, 38.1122) -> (7.347, 38.077) projected
  line L1444 (6.9471, 38.1222) -> (7.0016, 38.1122) projected
  line L1445 (6.8925, 38.1321) -> (6.9471, 38.1222) projected
  line L1446 (6.838, 38.1419) -> (6.8925, 38.1321) projected
  line L1447 (6.7834, 38.1516) -> (6.838, 38.1419) projected
  line L1448 (6.7289, 38.1613) -> (6.7834, 38.1516) projected
  line L1449 (6.6743, 38.1709) -> (6.7289, 38.1613) projected
  line L1450 (6.6197, 38.1804) -> (6.6743, 38.1709) projected
  line L1451 (6.5651, 38.1898) -> (6.6197, 38.1804) projected
  line L1452 (6.5105, 38.1992) -> (6.5651, 38.1898) projected
  line L1453 (6.4558, 38.2084) -> (6.5105, 38.1992) projected
  line L1454 (6.1191, 38.2935) -> (6.4558, 38.2084) projected
  line L1455 (5.8651, 38.3936) -> (6.1191, 38.2935) projected
  line L1456 (5.6532, 38.5075) -> (5.8651, 38.3936) projected
  line L1457 (5.4597, 38.636) -> (5.6532, 38.5075) projected
  line L1458 (5.2896, 38.7764) -> (5.4597, 38.636) projected
  line L1459 (5.1313, 38.9295) -> (5.2896, 38.7764) projected
  line L1460 (4.9918, 39.0931) -> (5.1313, 38.9295) projected
  line L1461 (4.8638, 39.2678) -> (4.9918, 39.0931) projected
  line L1462 (4.7503, 39.4526) -> (4.8638, 39.2678) projected
  line L1463 (4.6519, 39.6468) -> (4.7503, 39.4526) projected
  line L1464 (4.5622, 39.8511) -> (4.6519, 39.6468) projected
  line L1465 (4.4881, 40.0641) -> (4.5622, 39.8511) projected
  line L1466 (4.4278, 40.2859) -> (4.4881, 40.0641) projected
  line L1467 (4.3747, 40.5169) -> (4.4278, 40.2859) projected
  line L1468 (4.3353, 40.7562) -> (4.3747, 40.5169) projected
  line L1469 (4.3093, 41.0036) -> (4.3353, 40.7562) projected
  line L1470 (4.2964, 41.2588) -> (4.3093, 41.0036) projected
  line L1471 (4.291, 41.5224) -> (4.2964, 41.2588) projected
  line L1472 (4.2961, 41.7938) -> (4.291, 41.5224) projected
  line L1473 (4.3135, 42.0727) -> (4.2961, 41.7938) projected
  line L1474 (4.3176, 42.4502) -> (4.3135, 42.0727) projected
  line L1475 (4.294, 42.8304) -> (4.3176, 42.4502) projected
  line L1476 (4.2517, 43.2124) -> (4.294, 42.8304) projected
  line L1477 (4.1939, 43.5958) -> (4.2517, 43.2124) projected
  line L1478 (4.1223, 43.9802) -> (4.1939, 43.5958) projected
  line L1479 (4.0382, 44.3655) -> (4.1223, 43.9802) projected
  line L1480 (3.9425, 44.7515) -> (4.0382, 44.3655) projected
  line L1481 (3.8357, 45.1381) -> (3.9425, 44.7515) projected
  line L1482 (3.7184, 45.5251) -> (3.8357, 45.1381) projected
  line L1483 (3.591, 45.9125) -> (3.7184, 45.5251) projected
  line L1484 (3.4538, 46.3) -> (3.591, 45.9125) projected
  line L1485 (3.3071, 46.6876) -> (3.4538, 46.3) projected
  line L1486 (3.1511, 47.0752) -> (3.3071, 46.6876) projected
  line L1487 (2.9861, 47.4626) -> (3.1511, 47.0752) projected
  line L1488 (2.8122, 47.8499) -> (2.9861, 47.4626) projected
  line L1489 (2.6297, 48.2368) -> (2.8122, 47.8499) projected
  line L1490 (2.4385, 48.6232) -> (2.6297, 48.2368) projected
  line L1491 (2.2389, 49.0092) -> (2.4385, 48.6232) projected
  line L1492 (2.031, 49.3945) -> (2.2389, 49.0092) projected
  line L1493 (1.8149, 49.7791) -> (2.031, 49.3945) projected
  line L1494 (1.452, 49.791) -> (1.8149, 49.7791) projected
  line L1495 (1.0891, 49.8003) -> (1.452, 49.791) projected
  line L1496 (0.7261, 49.8069) -> (1.0891, 49.8003) projected
  line L1497 (0.363, 49.8108) -> (0.7261, 49.8069) projected
  line L1498 (0, 49.8122) -> (0.363, 49.8108) projected
  line L1499 (-0.363, 49.8108) -> (0, 49.8122) projected
  line L1500 (-0.7261, 49.8069) -> (-0.363, 49.8108) projected
  line L1501 (-1.0891, 49.8003) -> (-0.7261, 49.8069) projected
  line L1502 (-1.452, 49.791) -> (-1.0891, 49.8003) projected
  line L1503 (-1.8149, 49.7791) -> (-1.452, 49.791) projected
  line L1504 (-2.031, 49.3945) -> (-1.8149, 49.7791) projected
  line L1505 (-2.2389, 49.0092) -> (-2.031, 49.3945) projected
  line L1506 (-2.4385, 48.6232) -> (-2.2389, 49.0092) projected
  line L1507 (-2.6297, 48.2368) -> (-2.4385, 48.6232) projected
  line L1508 (-2.8122, 47.8499) -> (-2.6297, 48.2368) projected
  line L1509 (-2.9861, 47.4626) -> (-2.8122, 47.8499) projected
  line L1510 (-3.1511, 47.0752) -> (-2.9861, 47.4626) projected
  line L1511 (-3.3071, 46.6876) -> (-3.1511, 47.0752) projected
  line L1512 (-3.4538, 46.3) -> (-3.3071, 46.6876) projected
  line L1513 (-3.591, 45.9125) -> (-3.4538, 46.3) projected
  line L1514 (-3.7184, 45.5251) -> (-3.591, 45.9125) projected
  line L1515 (-3.8357, 45.1381) -> (-3.7184, 45.5251) projected
  line L1516 (-3.9425, 44.7515) -> (-3.8357, 45.1381) projected
  line L1517 (-4.0382, 44.3655) -> (-3.9425, 44.7515) projected
  line L1518 (-4.1223, 43.9802) -> (-4.0382, 44.3655) projected
  line L1519 (-4.1939, 43.5958) -> (-4.1223, 43.9802) projected
  line L1520 (-4.2517, 43.2124) -> (-4.1939, 43.5958) projected
  line L1521 (-4.294, 42.8304) -> (-4.2517, 43.2124) projected
  line L1522 (-4.3176, 42.4502) -> (-4.294, 42.8304) projected
  line L1523 (-4.3156, 42.2598) -> (-4.3176, 42.4502) projected
  line L1524 (-4.3156, 42.2598) -> (-9.1991, 59.2906) projected
  arc A4 (-9.1991, 59.2906) -> (-51.5273, 30.7399) centre (0, 0) ccw projected
  line L1525 (-51.5273, 30.7399) -> (-43.4223, 24.4075) projected
  circle A5 centre (0, 0) radius 4 projected
  line L1526 (-51.5273, 30.7399) -> (-43.4223, 24.4075) projected
  circle A6 centre (0, 0) radius 15
  line L1527 (-4.3156, 42.2598) -> (-3.0587, 37.8767)
  line L1528 (-43.4223, 24.4075) -> (-33.9728, 17.0249)
  line L1529 (13.2606, 7.0112) -> (-3.0587, 37.8767)
  line L1530 (-33.9728, 17.0249) -> (-11.4682, -9.6686)
  line L1531 (9.2822, -36.8489) -> (10.2968, -40.8767)
  line L1532 (11.6871, 36.1581) -> (-4.3156, 42.2598)
  arc A7 (-33.9728, 17.0249) -> (11.6871, 36.1581) centre (0, 0) ccw
  line L1533 (9.2822, -36.8489) -> (-11.4682, -9.6686)
  line L1534 (15.32, 47.3978) -> (11.6871, 36.1581)
  circle A8 centre (0, 0) radius 9.5
  point P0 (21.3296, 31.4491)
  dimension "d28" = 30
  dimension "d45" = 19
  constraints: 16 end point, 6 point on circle, 3 centre point, 3 coincident, 3 point on line, 2 tangent, 1 midpoint
  measures "d28" diameter of A6
  measures "d45" diameter of A8
extrude "押し出し5" cut sketch "スケッチ4" against normal blind 3 contours L0 L1528 A7 L1531 L673 L672 L671 L670 L669 L668 L667 L666 L665 L664 L663 L662 L661 L660 L659 L658 L657 L656 L655 L654 L653 L652 L651 L650 L649 L648 L647 L646 L645 L644 L643 L642 L641 L640 L639 L638 L637 L636 L635 L634 L633 L632 L631 L630 L629 L628 L627 L626 L625 L624 L623 L622 L621 L620 L619 L618 L617 L616 L615 L614 L613 L612 L611 L610 L609 L608 L607 L606 L605 L604 L603 L602 L601 L600 L599 L598 L597 L596 L595 L594 L593 L592 L591 L590 L589 L588 L587 L586 L585 L584 L583 L582 L581 L580 L579 L578 L577 L576 L575 L574 L573 L572 L571 L570 L569 L568 L567 L566 L565 L564 L563 L562 L561 L560 L559 L558 L557 L556 L555 L554 L553 L552 L551 L550 L549 L548 L547 L546 L545 L544 L543 L542 L541 L540 L539 L538 L537 L536 L535 L534 L533 L532 L531 L530 L529 L528 L527 L526 L525 L524 L523 L522 L521 L520 L519 L518 L517 L516 L515 L514 L513 L512 L511 L510 L509 L508 L507 L506 L505 L504 L503 L502 L501 L500 L499 L498 L497 L496 L495 L494 L493 L492 L491 L490 L489 L488 L487 L486 L485 L484 L483 L482 L481 L480 L479 L478 L477 L476 L475 L474 L473 L472 L471 L470 L469 L468 L467 L466 L465 L464 L463 L462 L461 L460 L459 L458 L457 L456 L455 L454 L453 L452 L451 L450 L449 L448 L447 L446 L445 L444 L443 L442 L441 L440 L439 L438 L437 L436 L435 L434 L433 L432 L431 L430 L429 L428 L427 L426 L425 L424 L423 L422 L421 L420 L419 L418 L417 L416 L415 L414 L413 L412 L411 L410 L409 L408 L407 L406 L405 L404 L403 L402 L401 L400 L399 L398 L397 L396 L395 L394 L393 L392 L391 L390 L389 L388 L387 L386 L385 L384 L383 L382 L381 L380 L379 L378 L377 L376 L375 L374 L373 L372 L371 L370 L369 L368 L367 L366 L365 L364 L363 L362 L361 L360 L359 L358 L357 L356 L355 L354 L353 L352 L351 L350 L349 L348 L347 L346 L345 L344 L343 L342 L341 L340 L339 L338 L337 L336 L335 L334 L333 L332 L331 L330 L329 L328 L327 L326 L325 L324 L323 L322 L321 L320 L319 L318 L317 L316 L315 L314 L313 L312 L311 L310 L309 L308 L307 L306 L305 L304 L303 L302 L301 L300 L299 L298 L297 L296 L295 L294 L293 L292 L291 L290 L289 L288 L287 L286 L285 L284 L283 L282 L281 L280 L279 L278 L277 L276 L275 L274 L273 L272 L271 L270 L269 L268 L267 L266 L265 L264 L263 L262 L261 L260 L259 L258 L257 L256 L255 L254 L253 L252 L251 L250 L249 L248 L247 L246 L245 L244 L243 L242 L241 L240 L239 L238 L237 L236 L235 L234 L233 L232 L231 L230 L229 L228 L227 L226 L225 L224 L223 L222 L221 L220 L219 L218 L217 L216 L215 L214 L213 L212 L211 L210 L209 L208 L207 L206 L205 L204 L203 L202 L201 L200 L199 L198 L197 L196 L195 L194 L193 L192 L191 L190 L189 L188 L187 L186 L185 L184 L183 L182 L181 L180 L179 L178 L177 L176 L175 L174 L173 L172 L171 L170 L169 L168 L167 L166 L165 L164 L163 L162 L161 L160 L159 L158 L157 L156 L155 L154 L153 L152 L151 L150 L149 L148 L147 L146 L145 L144 L143 L142 L141 L140 L139 L138 L137 L136 L135 L134 L133 L132 L131 L130 L129 L128 L127 L126 L125 L124 L123 L122 L121 L120 L119 L118 L117 L116 L115 L114 L113 L112 L111 L110 L109 L108 L107 L106 L105 L104 L103 L102 L101 L100 L99 L98 L97 L96 L95 L94 L93 L92 L91 L90 L89 L88 L87 L86 L85 L84 L83 L82 L81 L80 L79 L78 L77 L76 L75 L74 L73 L72 L71 L70 L69 L68 L67 L66 L65 L64 L63 L62 L61 L60 L59 L58 L57 L56 L55 L54 L53 L52 L51 L50 L49 L48 L47 L46 L45 L44 L43 L42 L41 L40 L39 L38 L37 L36 L35 L34 L33 L32 L31 L30 L29 L28 L27 L26 L25 L24 L23 L22 L21 L20 L19 L18 L17 L16 L15 L14 L13 L12 L11 L10 L9 L8 L7 L6 L5 L4 L3 L2 L1 | L1530 L1533 A7 | L1523 L1522 L1521 L1520 L1519 L1518 L1517 L1516 L1515 L1514 L1513 L1512 L1511 L1510 L1509 L1508 L1507 L1506 L1505 L1504 L1503 L1502 L1501 L1500 L1499 L1498 L1497 L1496 L1495 L1494 L1493 L1492 L1491 L1490 L1489 L1488 L1487 L1486 L1485 L1484 L1483 L1482 L1481 L1480 L1479 L1478 L1477 L1476 L1475 L1474 L1473 L1472 L1471 L1470 L1469 L1468 L1467 L1466 L1465 L1464 L1463 L1462 L1461 L1460 L1459 L1458 L1457 L1456 L1455 L1454 L1453 L1452 L1451 L1450 L1449 L1448 L1447 L1446 L1445 L1444 L1443 L1442 L1441 L1440 L1439 L1438 L1437 L1436 L1435 L1434 L1433 L1432 L1431 L1430 L1429 L1428 L1427 L1426 L1425 L1424 L1423 L1422 L1421 L1420 L1419 L1418 L1417 L1416 L1415 L1414 L1413 L1412 L1411 L1410 L1409 L1408 L1407 L1406 L1405 L1404 L1534 L1532 | A8